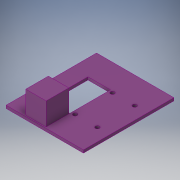
# Autodesk Inventor part: Sensor Board
Saved by Autodesk Inventor 2017 (Build 210142000, 142)
## iProperties
Created: 2017-02-20
Part Number: Sensor Board
Material: Generic
Document SubType Name: Modeling
Designer: qupec
Density: 1 g/cm^3
Appearance: Default
Author: qupec
Autodesk Inventor part; units mm, degrees
ref_plane "YZ Plane" through (0, 0, 0) normal (1, 0, 0) x (0, 1, 0)
sketch "Sketch1" plane through (0, 0, 0) normal (0, 1, 0) x (-1, 0, 0)
  line L0 (21.717, 25.4) -> (-21.717, 25.4)
  line L1 (-21.717, 25.4) -> (-21.717, -25.4)
  line L2 (-21.717, -25.4) -> (21.717, -25.4)
  line L3 (21.717, -25.4) -> (21.717, -11.43)
  line L4 (12.573, -11.43) -> (-0.127, -11.43)
  line L5 (-0.127, -11.43) -> (-0.127, 11.43)
  line L6 (-0.127, 11.43) -> (12.573, 11.43)
  line L7 (21.717, 11.43) -> (21.717, 25.4)
  line L8 (12.573, -11.43) -> (12.573, 11.43)
  line L9 (21.717, 11.43) -> (21.717, -11.43)
  point P0 (0, 0)
  dimension "d0" = 43.434
  dimension "d1" = 43.434
  dimension "d2" = 21.717
  dimension "d3" = 50.8
  dimension "d4" = 25.4
  dimension "d33" = 21.59
  dimension "d34" = 12.7
  dimension "d35" = 13.97
  dimension "d36" = 13.97
  constraints: 20 end point, 8 perpendicular, 1 horizontal
  measures "d0" distance between parallel lines of L1 L7
  measures "d1" distance between parallel lines of L1 L3
  measures "d2" distance from line of point (0, 0) L7
  measures "d3" distance between parallel lines of L2 L0
  measures "d4" distance from line of point (0, 0) L0
  measures "d33" distance between parallel lines of L5 L1
  measures "d34" distance between parallel lines of L8 L5
  measures "d35" distance between parallel lines of L2 L4
  measures "d36" distance between parallel lines of L0 L6
ref_plane "Work Plane2" through (0, 1.6, 0) normal (0, 1, 0) x (1, 0, 0)
extrude "Extrusion4" add sketch "Sketch1" along normal blind 1.6
ref_plane "Work Plane1" through (0, 1.6, 0) normal (0, 1, 0) x (1, 0, 0)
sketch "Sketch3" plane through (0, 1.6, 0) normal (0, 1, 0) x (1, 0, 0)
  circle A0 centre (2.1387, -10.5016) radius 1.143
  circle A1 centre (2.1387, 10.5016) radius 1.143
  circle A2 centre (14.638, -10.5016) radius 1.143
  circle A3 centre (14.638, 10.5016) radius 1.143
  line L0 (21.717, -25.4) -> (21.717, 25.4) projected
  point P0 (0, 0)
  dimension "d19" = 2.286
  dimension "d20" = 2.286
  dimension "d21" = 2.286
  dimension "d22" = 2.286
  dimension "d23" = 21.0033
  dimension "d24" = 21.0033
  dimension "d27" = 12.4993
  dimension "d30" = 12.4993
  dimension "d42" = 7.079
  dimension "d43" = 7.079
  dimension "d44" = 10.5016
  constraints: 4 centre point
  measures "d19" diameter of A0
  measures "d20" diameter of A1
  measures "d21" diameter of A2
  measures "d22" diameter of A3
  measures "d23" distance of A3.centre A2.centre
  measures "d24" distance of A1.centre A0.centre
  measures "d27" distance of A2.centre A0.centre
  measures "d30" distance of A3.centre A1.centre
  measures "d42" distance from line of L0 A3.centre
  measures "d43" distance from line of L0 A2.centre
  measures "d44" vertical distance of A0.centre point (0, 0)
extrude "Extrusion6" cut sketch "Sketch3" against normal through all
sketch "Sketch4" plane through (0, 1.6, 0) normal (0, 1, 0) x (1, 0, 0)
  line L0 (-11.303, -24.765) -> (0.127, -24.765)
  line L1 (0.127, -24.765) -> (0.127, -12.065)
  line L2 (0.127, -12.065) -> (-11.303, -12.065)
  line L3 (-11.303, -12.065) -> (-11.303, -24.765)
  line L4 (-12.573, -11.43) -> (-12.573, 11.43) projected
  line L5 (0.127, 11.43) -> (0.127, -11.43) projected
  line L6 (-21.717, -25.4) -> (21.717, -25.4) projected
  point P0 (0, 0)
  dimension "d48" = 0
  dimension "d49" = 11.43
  dimension "d50" = 12.7
  dimension "d51" = 0.635
  constraints: 8 end point, 2 parallel, 1 horizontal, 1 perpendicular
  measures "d48" distance between parallel lines of L5 L1
  measures "d49" distance between parallel lines of L1 L3
  measures "d50" distance between parallel lines of L0 L2
  measures "d51" distance between parallel lines of L6 L0
extrude "Extrusion7" add sketch "Sketch4" along normal blind 12.7
equation "\"d1\" = d0"
equation "\"d2\" = 0.5 * d0"
equation "\"d4\" = 0.5 * d3"
equation "\"d36\" = d35"
equation "\"d20\" = d19"
equation "\"d21\" = d20"
equation "\"d22\" = d21"
equation "\"d24\" = d23"
equation "\"d30\" = d27"
equation "\"d43\" = d42"
equation "\"d44\" = 0.5 * d24"
body "Solid1"
